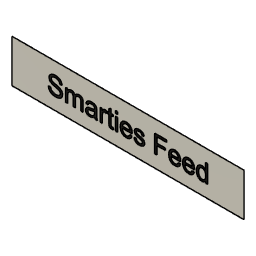
smartie_sorter_3000 (Autodesk Fusion 360 archive; units mm, degrees)
design "Smarties Feed Label"
part number: 2025-04-13-10-05-08-737
Autodesk Fusion 360 part; units mm, degrees
sketch "Sticker" plane through (0, 0, 0) normal (0, 1, 0) x (1, 0, 0)
  line L0 (0, 0) -> (65, 0)
  line L1 (65, 0) -> (65, -12)
  line L2 (65, -12) -> (0, -12)
  line L3 (0, -12) -> (0, 0)
  dimension "d1" = 12
  dimension "d2" = 65
  constraint horizontal L0
  constraint vertical L1
  constraint horizontal L2
  constraint vertical L3
  constraint coincident L0.start L3.end
  measures "d1" distance of L0.end L1.end
  measures "d2" distance of L0.start L0.end
extrude "Extrude1" add sketch "Sticker" along normal blind 0.01 makes body 1
sketch "Text" plane through (0, 0, 0) normal (0, -1, 0) x (1, 0, 0)
  line L0 (65, 12) -> (0, 12)
  line L1 (0, 12) -> (0, 0)
  line L2 (0, 0) -> (65, 0)
  line L3 (65, 0) -> (65, 12)
  line L4 (0, 0) -> (65, 0) construction
  line L5 (65, 0) -> (65, 12) construction
  line L6 (65, 12) -> (0, 12) construction
  line L7 (0, 12) -> (0, 0) construction
  dimension "d5" = 5
  text T0 "Smarties Feed" font "Arial" height 5 align centre middle in box 65 x 12 at (0, 0) x (1, 0) y (0, 1) spacing 1 kerned
  constraint coincident L2.end
  constraint coincident L0.end
extrude "Extrude2" add sketch "Text" along normal blind 0.01 separate body text T0 makes body 2 at (15.2098, 0, 5.3338) makes body 3 at (24.9062, 0, 5.3395) makes body 4 at (29.3878, 0, 8.0293) makes body 5 at (29.3878, 0, 4.7074) makes body 6 at (36.084, 0, 5.3662) makes body 7 at (46.1272, 0, 5.3224) makes body 8 at (50.0119, 0, 5.3224) makes body 9 at (40.1779, 0, 5.9238) makes body 10 at (32.5426, 0, 5.3224) makes body 11 at (54.6076, 0, 5.8807) makes body 12 at (27.554, 0, 5.244) makes body 13 at (23.5463, 0, 4.5282) makes body 14 at (12.6004, 0, 5.8956)
named bodies: "Sticker", "Text 2", "Text 4", "Text 7", "Text 6", "Text 9", "Text 11", "Text 12", "Text 10", "Text 8", "Text 13", "Text 5", "Text 3", "Text 1"

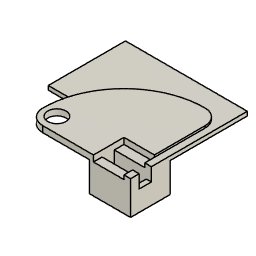
design "Colour Detection Mechanism Platform"
Autodesk Fusion 360 part; units mm, degrees
sketch "Colour Detection Mechanism Platform" plane through (0, 0, 0) normal (0, 0, 1) x (1, 0, 0)
  line L0 (0, 0) -> (120, 0)
  line L1 (120, 0) -> (120, 76)
  line L2 (120, 76) -> (0, 76)
  line L3 (0, 76) -> (0, 0)
  dimension "d169" = 120
  dimension "d170" = 76
  constraint horizontal L0
  constraint vertical L1
  constraint horizontal L2
  constraint vertical L3
  constraint coincident L0.start L3.end
  measures "d169" distance of L0.start L0.end
  measures "d170" distance of L0.start L2.end
extrude "Extrude42" add sketch "Colour Detection Mechanism Platform" along normal blind 4
sketch "Smartie Path" plane through (0, 0, 4) normal (0, 0, 1) x (-1, 0, 0)
  line L0 (0, -76) -> (0, 0)
  line L1 (0, 0) -> (-120, 0)
  line L2 (-120, 0) -> (-120, -76)
  line L3 (-120, -76) -> (0, -76)
  circle A0 centre (-98.5, 24) radius 80
  line L4 (-98.5, 24) -> (-113.5, 24)
  line L5 (-113.5, 24) -> (-113.5, -56)
  line L6 (-113.5, -56) -> (-98.5, -56)
  line L7 (-98.5, -56) -> (-98.5, 24)
  line L8 (-98.5, 24) -> (-18.5, 24)
  line L9 (-18.5, 24) -> (-18.5, 39)
  line L10 (-18.5, 39) -> (-98.5, 39)
  line L11 (-98.5, 39) -> (-98.5, 24)
  line L12 (-98.5, 24) -> (-113.5, 24)
  line L13 (-113.5, 24) -> (-113.5, 39)
  line L14 (-113.5, 39) -> (-98.5, 39)
  line L15 (-98.5, 39) -> (-98.5, 24)
  circle A1 centre (-32.5, 24) radius 9
  dimension "d173" = 160
  dimension "d174" = 24
  dimension "d175" = 21.5
  dimension "d176" = 15
  dimension "d177" = 15
  dimension "d178" = 80
  dimension "d179" = 80
  dimension "d184" = 18
  dimension "d185" = 14
  constraint horizontal L4
  constraint vertical L5
  constraint horizontal L6
  constraint vertical L7
  constraint coincident A0.centre L4.start
  constraint horizontal L8
  constraint vertical L9
  constraint horizontal L10
  constraint vertical L11
  constraint horizontal L12
  constraint vertical L13
  constraint horizontal L14
  constraint vertical L15
  constraint collinear L5 L13
  constraint collinear L10 L14
  constraint coincident L8 A1.centre
  measures "d173" diameter of A0
  measures "d174" distance of L1 A0.centre
  measures "d175" horizontal distance of L1.end A0.centre
  measures "d176" distance of L8.end L9.end
  measures "d177" distance of L5.end L6.end
  measures "d178" distance of L4.end L5.end
  measures "d179" distance of L9.end L10.end
  measures "d184" diameter of A1
  measures "d185" distance of L8.end A1.centre
extrude "Extrude43" add sketch "Smartie Path" along normal blind 2 contours L1 A0 L7 | L1 A0 L7 L8 A1 | L1 A0 L5 L7 | L1 L4 L5 L7 L12 | A0 L8 L10 L11 L15 A1 | L4 L11 L12 L13 L14 L15
fillet "Fillet2" radius 15 2 edges at (19.9188, -39, 5) (113.5, 54.5812, 5)
extrude "Extrude44" add 1 faces at (89.4665, -20.5529, 4) along direction (0, 0, -1) blind 4
sketch "Servo Hole" plane through (0, 0, 6) normal (0, 0, 1) x (-1, 0, 0)
  circle A0 centre (-32.5, 24) radius 9
  arc A1 (-113.5, -41) -> (-98.5, -56) centre (-98.5, -41) ccw
  arc A2 (-98.5, -56) -> (-18.5, 24) centre (-98.5, 24) ccw
  arc A3 (-18.5, 24) -> (-33.5, 39) centre (-33.5, 24) ccw
  line L0 (-33.5, 39) -> (-113.5, 39)
  line L1 (-113.5, 39) -> (-113.5, -41)
  line L2 (-113.5, 39) -> (-83.5, 39)
  line L3 (-83.5, 39) -> (-83.5, 9)
  line L4 (-83.5, 9) -> (-113.5, 9)
  line L5 (-113.5, 9) -> (-113.5, 39)
  dimension "d188" = 30
  dimension "d189" = 30
  constraint horizontal L2
  constraint vertical L3
  constraint horizontal L4
  constraint vertical L5
  constraint coincident L0.end L1.start
  measures "d188" distance of L3.end L4.end
  measures "d189" distance of L2.end L3.end
extrude "Extrude45" cut sketch "Servo Hole" against normal blind 6 contours L0 L1 L2 L3 L4 L5
sketch "Servo Holder" plane through (0, 0, 0) normal (0, 0, -1) x (1, 0, 0)
  line L0 (113.5, 9) -> (83.5, 9)
  line L1 (83.5, 9) -> (83.5, 39)
  line L2 (83.5, 39) -> (33.5, 39)
  arc A0 (33.5, 39) -> (18.5, 24) centre (33.5, 24) ccw
  arc A1 (18.5, 24) -> (22.1849, 0) centre (98.5, 24) ccw
  line L3 (22.1849, 0) -> (0, 0)
  line L4 (0, 0) -> (0, -76)
  line L5 (0, -76) -> (120, -76)
  line L6 (120, -76) -> (120, 0)
  line L7 (120, 0) -> (113.5, 0)
  line L8 (113.5, 0) -> (113.5, 9)
  circle A2 centre (32.5, 24) radius 9
  line L9 (120, 0) -> (79.5, 0)
  line L10 (79.5, 0) -> (79.5, 39)
  line L11 (79.5, 39) -> (120, 39)
  line L12 (120, 39) -> (120, 0)
  dimension "d192" = 40.5
  constraint horizontal L9
  constraint vertical L10
  constraint horizontal L11
  constraint vertical L12
  constraint coincident L6.end L7.start
  constraint collinear L2 L11
  measures "d192" distance of L10.end L11.end
extrude "Extrude46" add sketch "Servo Holder" along normal blind 29 contours L0 L1 L2 L8 L9 L10 L11 | L0 L1 L7 L8 L9 L11 L12
extrude "Extrude50" add 1 faces at (105.6667, -29, 0) along direction (0, 0, 1) blind 4
sketch "Servo Seat" plane through (0, 0, 4) normal (0, 0, 1) x (-1, 0, 0)
  line L0 (-113.5, -41) -> (-113.5, 9)
  line L1 (-113.5, 9) -> (-83.5, 9)
  line L2 (-83.5, 9) -> (-83.5, 39)
  line L3 (-83.5, 39) -> (-120, 39)
  line L4 (-120, 39) -> (-120, -76)
  line L5 (-120, -76) -> (0, -76)
  line L6 (0, -76) -> (0, 0)
  line L7 (0, 0) -> (-22.1849, 0)
  arc A0 (-98.5, -56) -> (-22.1849, 0) centre (-98.5, 24) ccw
  arc A1 (-113.5, -41) -> (-98.5, -56) centre (-98.5, -41) ccw
  line L8 (-83.5, 9) -> (-120, 9)
  line L9 (-120, 9) -> (-120, 18.5)
  line L10 (-120, 18.5) -> (-83.5, 18.5)
  line L11 (-83.5, 18.5) -> (-83.5, 9)
  line L12 (-83.5, 39) -> (-120, 39)
  line L13 (-120, 39) -> (-120, 30.5)
  line L14 (-120, 30.5) -> (-83.5, 30.5)
  line L15 (-83.5, 30.5) -> (-83.5, 39)
  line L16 (-120, 18.5) -> (-115, 18.5)
  line L17 (-115, 18.5) -> (-115, 30.5)
  line L18 (-115, 30.5) -> (-120, 30.5)
  line L19 (-120, 30.5) -> (-120, 18.5)
  line L20 (-113.5, 9) -> (-113.5, 18.5)
  line L21 (-113.5, 30.5) -> (-113.5, 39)
  dimension "d208" = 9.5
  dimension "d211" = 5
  dimension "d225" = 12
  dimension "d226" = 8.5
  dimension "d227" = 6.5
  constraint horizontal L8
  constraint vertical L9
  constraint horizontal L10
  constraint vertical L11
  constraint coincident L1.end L2.start
  constraint horizontal L12
  constraint vertical L13
  constraint horizontal L14
  constraint vertical L15
  constraint coincident L2.end L3.start
  constraint coincident L4 L9.end
  constraint horizontal L16
  constraint vertical L17
  constraint horizontal L18
  constraint vertical L19
  constraint coincident L14 L17.end
  constraint coincident L0.end L1.start
  constraint coincident L10 L20.end
  constraint perpendicular L10 L20
  constraint coincident L14 L21.start
  constraint coincident L3 L21.end
  constraint perpendicular L3 L21
  constraint collinear L20 L21
  constraint collinear L9 L13
  measures "d208" distance of L8.end L9.end
  measures "d211" distance of L17 L19
  measures "d225" distance of L9.end L13.end
  measures "d226" distance of L3.end L13.end
  measures "d227" distance of L13 L21
extrude "Extrude51" cut sketch "Servo Seat" against normal blind 13 contours L4 L10 L14 L16 L17 L18 L19
extrude "Extrude52" cut sketch "Servo Seat" against normal blind 4 contours L1 L2 L8 L10 L11 L20 | L2 L3 L12 L14 L15 L21
extrude "Extrude53" cut sketch "Servo Seat" against normal blind 29 contours L2 L10 L14 L17
sketch "Servo Wires Hole" plane through (79.5, 0, 0) normal (-1, 0, 0) x (0, -1, 0)
  line L0 (39, 0) -> (0, 0)
  line L1 (0, 0) -> (0, -29)
  line L2 (0, -29) -> (39, -29)
  line L3 (39, -29) -> (39, 0)
  line L4 (18.5, -15) -> (30.5, -15)
  line L5 (30.5, -15) -> (30.5, -25)
  line L6 (30.5, -25) -> (18.5, -25)
  line L7 (18.5, -25) -> (18.5, -15)
  dimension "d219" = 8.5
  dimension "d220" = 4
  dimension "d221" = 10
  dimension "d228" = 12
  constraint horizontal L4
  constraint vertical L5
  constraint horizontal L6
  constraint vertical L7
  measures "d219" distance of L3 L5
  measures "d220" distance of L2 L6
  measures "d221" distance of L4.end L5.end
  measures "d228" distance of L5.end L6.end
extrude "Extrude54" cut sketch "Servo Wires Hole" against normal blind 4 contours L4 L5 L6 L7
equation "d62 = 29.5 mm + 1 mm"
equation "d66 = 16.5 mm + 4 mm"
equation "d67 = ( 20.5 * 2 ) * 1 mm"
equation "d74 = ( ( 24 + 8.5 + 20 + 4 ) * 2 ) * 1 mm"
equation "d75 = 24 mm + 8.5 mm + 10 mm"
equation "d76 = ( ( 113 / 2 ) * 1 mm )"
equation "d77 = ( ( 113 / 2 ) * 1 mm )"
equation "d95 = 4 mm + 1.5 mm"
equation "d103 = -( 29 mm - 16 mm )"
named bodies: "Colour Detection Mechanism Platform"

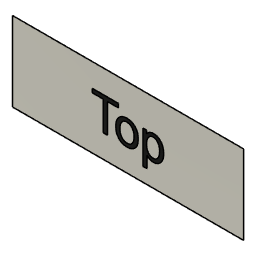
design "Top Label"
part number: 2025-04-13-09-56-45-957
Autodesk Fusion 360 part; units mm, degrees
sketch "Sticker" plane through (0, 0, 0) normal (0, 1, 0) x (1, 0, 0)
  line L0 (0, 0) -> (35, 0)
  line L1 (35, 0) -> (35, -12)
  line L2 (35, -12) -> (0, -12)
  line L3 (0, -12) -> (0, 0)
  dimension "d1" = 35
  dimension "d2" = 12
  constraint horizontal L0
  constraint vertical L1
  constraint horizontal L2
  constraint vertical L3
  constraint coincident L0.start L3.end
  measures "d1" distance of L0.start L0.end
  measures "d2" distance of L0.end L1.end
extrude "Extrude1" add sketch "Sticker" along normal blind 0.01 makes body 1
sketch "Text" plane through (0, 0, 0) normal (0, -1, 0) x (1, 0, 0)
  line L0 (35, 12) -> (0, 12)
  line L1 (0, 12) -> (0, 0)
  line L2 (0, 0) -> (35, 0)
  line L3 (35, 0) -> (35, 12)
  line L4 (0, 0) -> (35, 0) construction
  line L5 (35, 0) -> (35, 12) construction
  line L6 (35, 12) -> (0, 12) construction
  line L7 (0, 12) -> (0, 0) construction
  dimension "d5" = 5
  text T0 "Top" font "Arial" height 5 align centre middle in box 35 x 12 at (0, 0) x (1, 0) y (0, 1) spacing 1 kerned
  constraint coincident L2.end
  constraint coincident L0.end
extrude "Extrude2" add sketch "Text" along normal blind 0.01 separate body text T0 makes body 2 at (19.9566, 0, 4.7193) makes body 3 at (15.8803, 0, 5.5613) makes body 4 at (14.1792, 0, 4.97)
named bodies: "Sticker", "Text 3", "Text 2", "Text 1"
